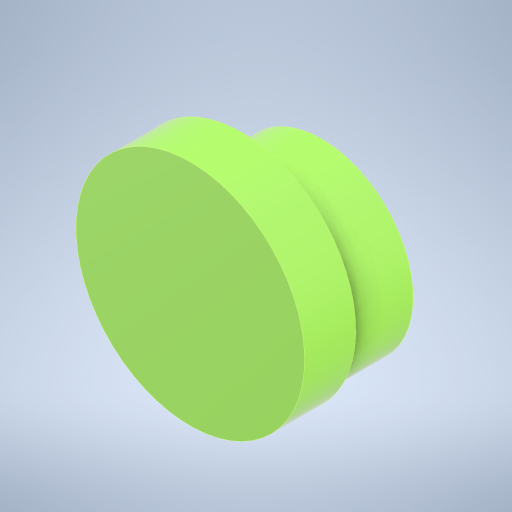
# Autodesk Inventor part: Back motor
Saved by Autodesk Inventor 2023 (Build 270158000, 158)
## iProperties
Created: 2022-05-02
Part Number: Back motor
Material: Phenolic Resin
Document SubType Name: Modeling
Designer: Devin
Density: 1.38 g/cm^3
Appearance: Light Green
Author: Devin
Autodesk Inventor part; units mm, degrees
ref_plane "YZ Plane" through (0, 0, 0) normal (1, 0, 0) x (0, 1, 0)
ref_plane "XZ Plane" through (0, 0, 0) normal (0, 1, 0) x (-1, 0, 0)
ref_plane "XY Plane" through (0, 0, 0) normal (0, 0, 1) x (1, 0, 0)
sketch "Sketch1" plane through (0, 0, 0) normal (0, 0, 1) x (1, 0, 0)
  circle A0 centre (0, 0) radius 5.08
  dimension "d0" = 10.16
  constraints: 1 centre point, 1 coincident
  measures "d0" diameter of A0
extrude "Extrusion1" add sketch "Sketch1" along normal blind 2.286
sketch "Sketch2" plane through (0, 0, 0) normal (0, 0, -1) x (-1, 0, 0)
  circle A0 centre (0, -1.016) radius 4.064
  circle A1 centre (0, 0) radius 5.08 projected
  dimension "d3" = 8.128
  constraints: 1 centre point, 1 tangent, 1 vertical alignment
  measures "d3" diameter of A0
extrude "Extrusion2" add sketch "Sketch2" along normal blind 3.556 contours A0
sketch "Sketch3" plane through (0, -1.016, -3.556) normal (0, 0, -1) x (-1, 0, 0)
  circle A0 centre (0, 1.016) radius 5.08 projected
  point P0 (0, -2.54)
  point P1 (0, -4.064)
  dimension "d6" = 1.524
  constraints: 1 vertical alignment, 1 other
  measures "d6" distance of point (0, -4.064) point (0, -2.54)
hole "Hole1" at (0, -3.556, -3.556) direction (0, 0, 1) diameter 1.524 depth 5.08 tip angle 118
sketch "Sketch4" plane through (0, -1.016, -3.556) normal (0, 0, -1) x (-1, 0, 0)
  circle A0 centre (0, 0.889) radius 1.905
  circle A1 centre (0, -2.54) radius 0.762 projected
  circle A2 centre (0, 0) radius 4.064 projected
  point P0 (0, 1.016)
  point P1 (0, -1.778)
  point P2 (0, 2.794)
  point P3 (0, 4.064)
  dimension "d14" = 3.81
  dimension "d16" = 1.27
  constraints: 3 vertical alignment, 4 other
  measures "d16" distance of point (0, 4.064) point (0, 2.794)
extrude "Extrusion3" cut sketch "Sketch4" against normal blind 3.048 contours A0
body "Solid1"
